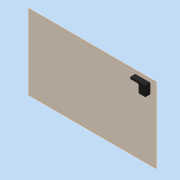
# Autodesk Inventor part: Part69
Saved by Autodesk Inventor 2017 (Build 210142000, 142)
## iProperties
Created: 2018-10-05
Part Number: Part69
Material: ABS Plastic
Document SubType Name: Modeling
Designer: mailb
Density: 1.06 g/cm^3
Appearance: Asphalt 2
Author: mailb
Autodesk Inventor part; units mm, degrees
ref_plane "YZ Plane" through (0, 0, 0) normal (1, 0, 0) x (0, 1, 0)
ref_plane "XZ Plane" through (0, 0, 0) normal (0, 1, 0) x (-1, 0, 0)
ref_plane "XY Plane" through (0, 0, 0) normal (0, 0, 1) x (1, 0, 0)
ref_plane "Work Plane1" through (0, 0, 0) normal (0, 0, 1) x (1, 0, 0)
sketch "Sketch1" plane through (0, 0, 0) normal (0, 0, 1) x (1, 0, 0)
  line L0 (254.7, 154.94) -> (254.7, 140.97) projected
  line L1 (254.7, -154.94) -> (254.7, 140.97) projected
  arc A0 (254.7, 154.94) -> (250.89, 158.75) centre (250.89, 154.94) ccw projected
  line L2 (-274.89, 158.75) -> (250.89, 158.75) projected
  arc A1 (260.25, -24.13) -> (261.52, -25.4) centre (261.52, -24.13) ccw projected
  line L3 (260.25, -24.13) -> (260.25, -21.59) projected
  arc A2 (261.52, -20.32) -> (260.25, -21.59) centre (261.52, -21.59) ccw projected
  line L4 (261.52, -20.32) -> (265.66, -20.32) projected
  arc A3 (266.93, -21.59) -> (265.66, -20.32) centre (265.66, -21.59) ccw projected
  line L5 (266.93, -21.59) -> (266.93, -24.13) projected
  arc A4 (265.66, -25.4) -> (266.93, -24.13) centre (265.66, -24.13) ccw projected
  line L6 (265.66, -25.4) -> (261.52, -25.4) projected
  arc A5 (-288.0375, 171.2625) -> (-291.2125, 168.0875) centre (-288.0375, 168.0875) ccw projected
  line L7 (-291.2125, -168.0875) -> (-291.2125, 168.0875) projected
  arc A6 (-291.2125, -168.0875) -> (-288.0375, -171.2625) centre (-288.0375, -168.0875) ccw projected
  line L8 (288.0375, -171.2625) -> (-288.0375, -171.2625) projected
  arc A7 (288.0375, -171.2625) -> (291.2125, -168.0875) centre (288.0375, -168.0875) ccw projected
  line L9 (291.2125, 168.0875) -> (291.2125, -168.0875) projected
  arc A8 (291.2125, 168.0875) -> (288.0375, 171.2625) centre (288.0375, 168.0875) ccw projected
  line L10 (-288.0375, 171.2625) -> (288.0375, 171.2625) projected
  circle A9 centre (264.3, 19.25) radius 3.6 projected
  line L11 (295.2621, 171.2883) -> (295.2621, 171.2625)
  line L12 (291.2125, 120.65) -> (254.7, 120.65)
  line L13 (215.0125, 171.2625) -> (215.0125, 158.75)
  point P0 (0, 0)
  constraints: 6 end point, 5 point on line, 1 perpendicular, 1 vertical
extrude "Extrusion1" add sketch "Sketch1" along normal blind 25.4 contours A0 L2 L13 L10 A8 L9 L12 L1 L0
chamfer "Chamfer1" distance 3.175 angle 45 3 edges at (254.7, 130.81, 25.4) (253.5841, 157.6341, 25.4) (232.9512, 158.75, 25.4)
body "Solid1"
